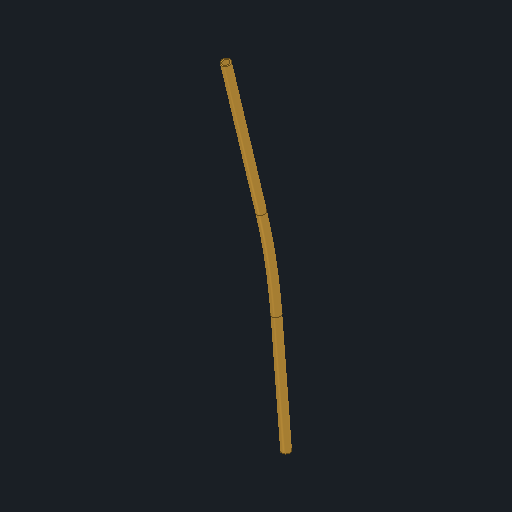
# Autodesk Inventor part: prop_shaft
Saved by Autodesk Inventor 2023 (Build 270158030, 158C)
## iProperties
Created: 2022-04-18
Part Number: prop_shaft
Material: Generic
Document SubType Name: Modeling
Designer: kardo
Density: 1 g/cm^3
Appearance: Brass - Prop shaft
Mass: 2.97565 g
Surface Area: 75.2146 cm^2
Volume: 2.97565 cm^3
Author: kardo
Autodesk Inventor part; units mm, degrees
ref_plane "YZ Plane" through (0, 0, 0) normal (1, 0, 0) x (0, 1, 0)
ref_plane "XZ Plane" through (0, 0, 0) normal (0, 1, 0) x (-1, 0, 0)
ref_plane "XY Plane" through (0, 0, 0) normal (0, 0, 1) x (1, 0, 0)
derived "stencil_frame.ipt"
sketch "sk_drivetrain_profile" plane through (6, 0, 0) normal (1, 0, 0) x (0, 1, 0)
  line L0 (-529.1844, 0) -> (410.1064, 0) construction
  line L1 (-345, 3089.1136) -> (-345, -1866.0023) construction
  line L2 (0, 3089.1136) -> (0, -1866.0023) construction
  line L3 (-140.3859, 53.0487) -> (-133.8494, 25.8223)
  line L4 (-377, 0) -> (-313.1973, 5.0214)
  line L5 (-137.1176, 39.4355) -> (-233.3061, 16.3427)
  line L6 (-296.4782, 6.3372) -> (-264.4984, 8.8541) construction
  line L7 (-264.4984, 8.8541) -> (-233.3061, 16.3427) construction
  line L8 (-133.8494, 25.8223) -> (-133.8494, 20.8223) construction
  line L9 (-313.1973, 5.0214) -> (-296.4782, 6.3372)
  line L10 (-850.7464, 3011.9134) -> (325.2296, -1886.3794) construction
  line L11 (-233.9547, 19.044) -> (-137.7662, 42.1369) construction
  line L12 (-136.4691, 36.7341) -> (-232.6576, 13.6413) construction
  line L13 (-233.9547, 19.044) -> (-232.6576, 13.6413) construction
  spline S0 degree 2 poles (-296.4782, 6.3372) (-264.4984, 8.8541) (-233.3061, 16.3427) knots 1 1 1 2 2 2
  line L14 (0, 21.3303) -> (-241.5001, 18.9703) construction
  line L15 (-55.7851, 21.5852) -> (-309.9218, 19.1017) construction
  point P0 (0, 0)
  point P1 (-221.5492, 19.1653)
  point P2 (-209.1437, 19.2865)
  point P3 (-205.6699, 20.1205)
ref_plane "plane_motor_mount" through (0, -127.65, 0) normal (0, 0.9723699, 0.2334454) x (-1, 0, 0)
sketch "sk_prop_shaft_profile" plane through (0, -127.65, 0) normal (0, 0.9723699, 0.2334454) x (-1, 0, 0)
  circle A0 centre (-6, 40.5561) radius 2.7781
  point P0 (0, -29.7993)
  dimension "d1" = 5.5563
  constraints: 1 centre point, 1 coincident
  measures "d1" diameter of A0
derived "parameters_powertrain.ipt"
sweep "Sweep1" add profiles "sk_prop_shaft_profile" path "sk_drivetrain_profile" path curves L5 S0 L9 L4
shell "Shell1" thickness 0.7937 removed faces 2 at (5.8387, -377.04, 0.5088) at (6.6932, -137.261, 40.0326)
equation "\"d1\" = prop_shaft_sleeve_od"
equation "\"prop_shaft_sleeve_od\" = 5.55625"
body "Solid1"
